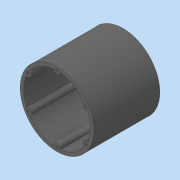
# Autodesk Inventor part: Spool
Saved by Autodesk Inventor 2017 (Build 210142000, 142)
## iProperties
Created: 2016-11-06
Part Number: Spool
Material: ABS Plastic
Document SubType Name: Modeling
Designer: techn
Density: 1.06 g/cm^3
Appearance: Gray
Author: techn
Autodesk Inventor part; units mm, degrees
ref_plane "YZ Plane" through (0, 0, 0) normal (1, 0, 0) x (0, 1, 0)
ref_plane "XZ Plane" through (0, 0, 0) normal (0, 1, 0) x (-1, 0, 0)
ref_plane "XY Plane" through (0, 0, 0) normal (0, 0, 1) x (1, 0, 0)
sketch "Sketch1" plane through (0, 0, 0) normal (0, 0, 1) x (1, 0, 0)
  circle A0 centre (0, 0) radius 33.655
  circle A1 centre (0, 0) radius 30.48
  dimension "d0" = 67.31
  dimension "d1" = 60.96
  constraints: 2 centre point, 2 coincident
  measures "d0" diameter of A0
  measures "d1" diameter of A1
extrude "Extrusion1" add sketch "Sketch1" along normal blind 60.325
sketch "Sketch3" plane through (0, 0, 60.325) normal (0, 0, 1) x (1, 0, 0)
  line L0 (0, 0) -> (0, 30.48)
  circle A0 centre (0, 30.48) radius 1.27
  circle A1 centre (0, 30.48) radius 3.175
  circle A2 centre (-26.3965, 15.24) radius 3.175
  circle A3 centre (-26.3965, 15.24) radius 1.27
  circle A4 centre (-26.3965, -15.24) radius 3.175
  circle A5 centre (-26.3965, -15.24) radius 1.27
  circle A6 centre (0, -30.48) radius 3.175
  circle A7 centre (0, -30.48) radius 1.27
  circle A8 centre (26.3965, -15.24) radius 3.175
  circle A9 centre (26.3965, -15.24) radius 1.27
  circle A10 centre (26.3965, 15.24) radius 3.175
  circle A11 centre (26.3965, 15.24) radius 1.27
  dimension "d4" = 30.48
  dimension "d5" = 2.54
  dimension "d6" = 6.35
  dimension "d9" = 360
  constraints: 12 centre point, 7 coincident, 2 end point, 1 vertical, 25 other
  measures "d4" distance of L0.start L0.end
  measures "d5" diameter of A0
  measures "d6" diameter of A1
extrude "Extrusion2" add sketch "Sketch3" against normal up to surface (60.325 mm away)
extrude "Extrusion3" cut sketch "Sketch3" against normal up to surface (60.325 mm away) contours A0 | A3 | A5 | A7 | A9 | A11
body "Solid1"
